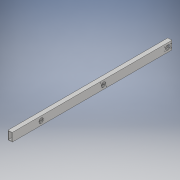
# Autodesk Inventor part: 41.75in Arm Beam Alternate (Right)
Saved by Autodesk Inventor 2018 (Build 220112000, 112)
## iProperties
Created: 2019-01-17
Part Number: 41.75in Arm Beam Alternate (Right)
Material: Generic
Document SubType Name: Modeling
Designer: Gabriel
Density: 1 g/cm^3
Appearance: Default
Author: Gabriel
Autodesk Inventor part; units mm, degrees
ref_plane "YZ Plane" through (0, 0, 0) normal (1, 0, 0) x (0, 1, 0)
ref_plane "XZ Plane" through (0, 0, 0) normal (0, 1, 0) x (-1, 0, 0)
ref_plane "XY Plane" through (0, 0, 0) normal (0, 0, 1) x (1, 0, 0)
sketch "Sketch1" plane through (0, 0, 0) normal (0, 0, 1) x (1, 0, 0)
  line L0 (-35.3228, 16.049) -> (-9.9228, 16.049)
  line L1 (-9.9228, 16.049) -> (-9.9228, -34.751)
  line L2 (-9.9228, -34.751) -> (-35.3228, -34.751)
  line L3 (-35.3228, -34.751) -> (-35.3228, 16.049)
  line L4 (-13.0978, 12.874) -> (-32.1478, 12.874)
  line L5 (-32.1478, 12.874) -> (-32.1478, -31.576)
  line L6 (-32.1478, -31.576) -> (-13.0978, -31.576)
  line L7 (-13.0978, -31.576) -> (-13.0978, 12.874)
  point P0 (0, 0)
  dimension "d0" = 25.4
  dimension "d1" = 50.8
  dimension "d2" = 3.175
  constraints: 16 end point, 4 parallel, 2 perpendicular, 1 horizontal, 3 other
  measures "d0" distance of L1.end L2.end
  measures "d1" distance of L0.end L1.end
  measures "d2" distance between parallel lines of L0 L4
extrude "Extrusion1" add sketch "Sketch1" along normal blind 977.9
sketch "Sketch2" plane through (-35.3228, -34.751, 0) normal (-1, 0, 0) x (0, 0, 1)
  line L0 (0, 0) -> (0, 50.8) construction
  line L1 (0, 25.4) -> (25.4, 25.4) construction
  circle A0 centre (25.4, 25.4) radius 12.7
  point P0 (0, 34.751)
  dimension "d5" = 25.4
  dimension "d9" = 25.4
  constraints: 2 end point, 1 centre point, 1 coincident, 1 horizontal, 1 midpoint
  measures "d5" distance of L1.start L1.end
  measures "d9" diameter of A0
extrude "Extrusion2" cut sketch "Sketch2" against normal blind 12.7
sketch "Sketch3" plane through (-35.3228, -34.751, 0) normal (-1, 0, 0) x (0, 0, 1)
  line L0 (977.9, 50.8) -> (977.9, 0) construction
  line L1 (977.9, 25.4) -> (800.1, 25.4) construction
  circle A0 centre (800.1, 25.4) radius 14.2875
  point P0 (0, 34.751)
  dimension "d10" = 177.8
  dimension "d11" = 28.575
  constraints: 2 end point, 1 centre point, 1 coincident, 1 horizontal, 1 midpoint
  measures "d10" distance of L1.start L1.end
  measures "d11" diameter of A0
extrude "Extrusion3" cut sketch "Sketch3" against normal blind 25.4
sketch "Sketch4" plane through (-35.3228, -34.751, 0) normal (-1, 0, 0) x (0, 0, 1)
  line L0 (977.9, 50.8) -> (977.9, 0) construction
  line L1 (977.9, 25.4) -> (419.1, 25.4) construction
  circle A0 centre (419.1, 25.4) radius 14.2875
  point P0 (0, 34.751)
  dimension "d14" = 558.8
  dimension "d15" = 28.575
  constraints: 2 end point, 1 centre point, 1 coincident, 1 horizontal, 1 midpoint
  measures "d14" distance of L1.start L1.end
  measures "d15" diameter of A0
extrude "Extrusion4" cut sketch "Sketch4" against normal blind 25.4
sketch "Sketch5" plane through (-35.3228, -34.751, 0) normal (-1, 0, 0) x (0, 0, 1)
  circle A0 centre (419.1, 25.4) radius 14.2875 construction
  line L0 (419.1, 25.4) -> (401.1395, 7.4395) construction
  line L1 (419.1, 25.4) -> (444.5, 25.4) construction
  line L2 (419.1, 25.4) -> (437.0605, 43.3605) construction
  circle A1 centre (401.1395, 7.4395) radius 2.032
  circle A2 centre (437.0605, 43.3605) radius 2.032
  point P0 (0, 34.751)
  dimension "d18" = 25.4
  dimension "d19" = 135
  dimension "d20" = 25.4
  dimension "d21" = 4.064
  dimension "d22" = 4.064
  constraints: 6 end point, 2 centre point, 2 coincident, 1 equal length, 1 horizontal
  measures "d18" distance of L0.start L0.end
  measures "d19" angle of L0 L1
  measures "d20" distance of L0.start L2.end
  measures "d21" diameter of A1
  measures "d22" diameter of A2
extrude "Extrusion5" cut sketch "Sketch5" against normal blind 25.4
sketch "Sketch6" plane through (-35.3228, -34.751, 0) normal (-1, 0, 0) x (0, 0, 1)
  line L0 (0, 47.625) -> (977.9, 47.625) projected
  circle A0 centre (25.4, 25.4) radius 12.7 projected
  line L1 (25.4482, 47.625) -> (44.6715, 36.4707)
  line L2 (44.6715, 36.4707) -> (44.6233, 14.2457)
  line L3 (44.6233, 14.2457) -> (25.3518, 3.175)
  line L4 (25.3518, 3.175) -> (6.1285, 14.3293)
  line L5 (6.1285, 14.3293) -> (6.1767, 36.5543)
  line L6 (6.1767, 36.5543) -> (25.4482, 47.625)
  circle A1 centre (44.6715, 36.4707) radius 2.5797
  circle A2 centre (44.6233, 14.2457) radius 2.5797
  circle A3 centre (6.1285, 14.3293) radius 2.5797
  circle A4 centre (6.1767, 36.5543) radius 2.5797
  dimension "d39" = 5.1594
  dimension "d40" = 5.1594
  dimension "d41" = 5.1594
  dimension "d42" = 5.1594
  constraints: 12 end point, 5 coincident, 4 centre point, 1 point on line, 13 other
  measures "d39" diameter of A1
  measures "d40" diameter of A2
  measures "d41" diameter of A3
  measures "d42" diameter of A4
sketch "Sketch7" plane through (-9.9228, -34.751, 0) normal (1, 0, 0) x (0, 0, -1)
  line L0 (0, 0) -> (0, 50.8) construction
  line L1 (0, 25.4) -> (-25.4, 25.4) construction
  circle A0 centre (-25.4, 25.4) radius 14.2875
  point P0 (0, 34.751)
  dimension "d34" = 25.4
  dimension "d35" = 28.575
  constraints: 2 end point, 1 centre point, 1 coincident, 1 horizontal, 1 midpoint
  measures "d34" distance of L1.start L1.end
  measures "d35" diameter of A0
extrude "Extrusion7" cut sketch "Sketch7" against normal blind 12.7
extrude "Extrusion8" cut sketch "Sketch6" against normal blind 25.4 contours A1 L2 L1 | L1 L2 A1 | A4 L5 L6 | L6 L5 A4 | A2 L3 L2 | L2 L3 A2 | A3 L4 L5 | L5 L4 A3
body "Solid1"
